Switch (Autodesk Fusion 360 design; units mm, degrees)
Autodesk Fusion 360 part; units mm, degrees
sketch "Sketch1" plane through (0, 0, 0) normal (0, 0, 1) x (1, 0, 0)
  line L0 (6.25, 9.25) -> (-6.25, 9.25)
  line L1 (-6.25, 9.25) -> (-6.25, -9.25)
  line L2 (-6.25, -9.25) -> (6.25, -9.25)
  line L3 (6.25, -9.25) -> (6.25, 9.25)
  line L4 (6.25, 9.25) -> (-6.25, -9.25) construction
  line L5 (-6.25, 9.25) -> (6.25, -9.25) construction
  dimension "d1" = 12.5
  dimension "d2" = 18.5
  constraint horizontal L0
  constraint perpendicular L0 L1
  constraint parallel L0 L2
  constraint parallel L1 L3
  constraint coincident L4 origin
  constraint coincident L5 origin
  measures "d1" distance of L1.end L2.end
  measures "d2" distance of L0.end L1.end
extrude "Extrude1" add sketch "Sketch1" along normal blind 10 makes body 1
sketch "Sketch2" plane through (0, 0, 10) normal (0, 0, 1) x (-1, 0, 0)
  line L0 (-6.25, 9.25) -> (-6.25, -9.25)
  line L1 (-6.25, -9.25) -> (6.25, -9.25)
  line L2 (6.25, -9.25) -> (6.25, 9.25)
  line L3 (6.25, 9.25) -> (-6.25, 9.25)
  line L4 (-6.5, -10) -> (6.5, -10)
  line L5 (6.5, -10) -> (6.5, 10)
  line L6 (6.5, 10) -> (-6.5, 10)
  line L7 (-6.5, 10) -> (-6.5, -10)
  line L8 (-6.5, -10) -> (6.5, 10) construction
  line L9 (6.5, -10) -> (-6.5, 10) construction
  dimension "d5" = 13
  dimension "d6" = 20
  constraint horizontal L4
  constraint perpendicular L4 L5
  constraint parallel L4 L6
  constraint parallel L5 L7
  constraint coincident L8 origin
  constraint coincident L9 origin
  measures "d5" distance of L5.end L6.end
  measures "d6" distance of L4.end L5.end
extrude "Extrude2" add sketch "Sketch2" along normal blind 4.5 contours L0 L1 L2 L3 | L4 L5 L6 L7 bodies 1
sketch "Sketch3" plane through (0, 0, 14.5) normal (0, 0, 1) x (-1, 0, 0)
  line L0 (-6.5, 10) -> (-6.5, -10)
  line L1 (-6.5, -10) -> (6.5, -10)
  line L2 (6.5, -10) -> (6.5, 10)
  line L3 (6.5, 10) -> (-6.5, 10)
  line L4 (-7.5, -10.5) -> (7.5, -10.5)
  line L5 (7.5, -10.5) -> (7.5, 10.5)
  line L6 (7.5, 10.5) -> (-7.5, 10.5)
  line L7 (-7.5, 10.5) -> (-7.5, -10.5)
  line L8 (-7.5, -10.5) -> (7.5, 10.5) construction
  line L9 (7.5, -10.5) -> (-7.5, 10.5) construction
  dimension "d9" = 15
  dimension "d10" = 21
  constraint horizontal L4
  constraint perpendicular L4 L5
  constraint parallel L4 L6
  constraint parallel L5 L7
  constraint coincident L8 origin
  constraint coincident L9 origin
  measures "d9" distance of L5.end L6.end
  measures "d10" distance of L4.end L5.end
extrude "Extrude3" add sketch "Sketch3" along normal blind 2 contours L0 L1 L2 L3 | L4 L5 L6 L7 bodies 1
sketch "Sketch4" plane through (0, 0, 16.5) normal (0, 0, 1) x (-1, 0, 0)
  line L0 (-7.5, 10.5) -> (-7.5, -10.5)
  line L1 (-7.5, -10.5) -> (7.5, -10.5)
  line L2 (7.5, -10.5) -> (7.5, 10.5)
  line L3 (7.5, 10.5) -> (-7.5, 10.5)
  line L4 (-5, -7.5) -> (5, -7.5)
  line L5 (5, -7.5) -> (5, 7.5)
  line L6 (5, 7.5) -> (-5, 7.5)
  line L7 (-5, 7.5) -> (-5, -7.5)
  line L8 (-5, -7.5) -> (5, 7.5) construction
  line L9 (5, -7.5) -> (-5, 7.5) construction
  dimension "d13" = 10
  dimension "d14" = 15
  constraint horizontal L4
  constraint perpendicular L4 L5
  constraint parallel L4 L6
  constraint parallel L5 L7
  constraint coincident L8 origin
  constraint coincident L9 origin
  measures "d13" distance of L5.end L6.end
  measures "d14" distance of L4.end L5.end
extrude "Extrude4" add sketch "Sketch4" along normal blind 3.5 contours L4 L5 L6 L7 bodies 1
sketch "Sketch5" plane through (5, 0, 0) normal (1, 0, 0) x (0, 1, 0)
  line L0 (-7.5, 16.5) -> (7.5, 16.5)
  line L1 (7.5, 16.5) -> (7.5, 20)
  line L2 (7.5, 20) -> (-7.5, 20)
  line L3 (-7.5, 20) -> (-7.5, 16.5)
  line L4 (0, 16.5) -> (7.5, 16.5)
  line L5 (0, 16.5) -> (-6.6332, 20)
  line L6 (-6.6332, 20) -> (-7.5, 16.5)
  dimension "d17" = 7.5
  constraint midpoint L0 L4.start
  constraint coincident L0.end L1.start
  constraint coincident L2 L5.end
  constraint coincident L0.start L3.end
  measures "d17" distance of L4.start L5.end
extrude "Extrude5" cut sketch "Sketch5" against normal blind 10 contours L2 L3 L6 | L0 L1 L2 L4 L5 bodies 1
sketch "Sketch6" plane through (0, 0, 16.5) normal (0, 0, 1) x (-1, 0, 0)
  line L0 (-5, 7.5) -> (5, 7.5)
  line L1 (5, 7.5) -> (5, 0)
  line L2 (5, 0) -> (-5, 0)
  line L3 (-5, 0) -> (-5, 7.5)
  line L4 (-7.5, 10.5) -> (-7.5, -10.5)
  line L5 (-7.5, -10.5) -> (7.5, -10.5)
  line L6 (7.5, -10.5) -> (7.5, 10.5)
  line L7 (7.5, 10.5) -> (-7.5, 10.5)
  line L8 (-5, -7.5) -> (5, -7.5)
  line L9 (5, -7.5) -> (5, 7.5)
  line L10 (5, 7.5) -> (-5, 7.5)
  line L11 (-5, 7.5) -> (-5, -7.5)
  line L12 (-5, -7.5) -> (5, 7.5) construction
  line L13 (5, -7.5) -> (-5, 7.5) construction
  line L14 (5.5, 8) -> (-5.5, 8)
  line L15 (-5.5, 8) -> (-5.5, -8)
  line L16 (-5.5, -8) -> (5.5, -8)
  line L17 (5.5, -8) -> (5.5, 8)
  dimension "d20" = 10
  dimension "d21" = 15
  dimension "d22" = 0.5
  constraint horizontal L8
  constraint perpendicular L8 L9
  constraint parallel L8 L10
  constraint parallel L9 L11
  constraint coincident L12 origin
  constraint coincident L13 origin
  measures "d20" distance of L0.end L0.start
  measures "d21" distance of L8.end L0.end
extrude "Extrude6" cut sketch "Sketch6" against normal blind 4 contours L14 L15 L16 L17 bodies 1
fillet "Fillet1" radius 1.5 4 edges at (7.5, -10.5, 15.5) (-7.5, -10.5, 15.5) (-7.5, 10.5, 15.5) (7.5, 10.5, 15.5) on bodies 1
fillet "Fillet2" radius 0.5 8 edges at (-7.0607, 10.0607, 16.5) (-7.5, 0, 16.5) (-7.0607, -10.0607, 16.5) (0, -10.5, 16.5) (7.0607, -10.0607, 16.5) (7.5, 0, 16.5) (7.0607, 10.0607, 16.5) (0, 10.5, 16.5) on bodies 1
fillet "Fillet3" radius 10 1 edges at (0, 0, 16.5) on bodies 1
fillet "Fillet4" radius 0.5 2 edges at (0, 7.5, 16.5) (0, -6.6332, 20) on bodies 1
fillet "Fillet5" radius 0.5 14 edges at (-5, -7.1434, 17.9399) (-5, -6.506, 19.7159) (-5, -4.1292, 18.6788) (-5, 0.0726, 16.7932) (-5, 4.7382, 16.5) (-5, 7.3536, 16.3536) (-5, 7.5, 14.25) (5, 7.5, 14.25) (5, 7.3536, 16.3536) (5, 4.7382, 16.5) (5, 0.0726, 16.7932) (5, -4.1292, 18.6788) (5, -6.506, 19.7159) (5, -7.1434, 17.9399) on bodies 1
sketch "Sketch7" plane through (0, 0, 16.5) normal (0, 0, 1) x (-1, 0, 0)
  line L0 (-4.5, -2.4764) -> (-4.5, -7)
  line L1 (-4.5, -7) -> (4.5, -7)
  line L2 (4.5, -7) -> (4.5, -2.4764)
  line L3 (4.5, -2.4764) -> (-4.5, -2.4764)
  line L4 (-4.5, -7) -> (4.5, -2.4764) construction
  circle A0 centre (0, -4.7382) radius 1.5
  dimension "d35" = 3
  constraint coincident L0.end L1.start
  constraint coincident L2.end L3.start
  constraint midpoint L4 A0.centre
  measures "d35" diameter of A0
extrude "Extrude7" add sketch "Sketch7" along normal blind 0.5 draft -45 contours A0 bodies 1
fillet "Fillet6" radius 0.5 1 edges at (0.9323, 4.3766, 17) on bodies 1
sketch "Sketch8" plane through (0, 0, 0) normal (0, 0, -1) x (1, 0, 0)
  line L0 (6.25, -9.25) -> (6.25, 9.25)
  line L1 (6.25, 9.25) -> (-6.25, 9.25)
  line L2 (-6.25, 9.25) -> (-6.25, -9.25)
  line L3 (-6.25, -9.25) -> (6.25, -9.25)
  line L4 (2.5, 7.5) -> (-2.5, 7.5) construction
  line L5 (-2.5, 7.5) -> (-2.5, -7.5) construction
  line L6 (-2.5, -7.5) -> (2.5, -7.5) construction
  line L7 (2.5, -7.5) -> (2.5, 7.5) construction
  line L8 (2.5, 7.5) -> (-2.5, -7.5) construction
  line L9 (-2.5, 7.5) -> (2.5, -7.5) construction
  line L10 (-2.5, 7.5) -> (2.5, 7.5)
  line L11 (2.5, 7.5) -> (2.5, 6.5)
  line L12 (2.5, 6.5) -> (-2.5, 6.5)
  line L13 (-2.5, 6.5) -> (-2.5, 7.5)
  line L14 (-2.5, -7.5) -> (2.5, -7.5)
  line L15 (2.5, -7.5) -> (2.5, -6.5)
  line L16 (2.5, -6.5) -> (-2.5, -6.5)
  line L17 (-2.5, -6.5) -> (-2.5, -7.5)
  line L18 (2.5, 0.5) -> (-2.5, 0.5)
  line L19 (-2.5, 0.5) -> (-2.5, -0.5)
  line L20 (-2.5, -0.5) -> (2.5, -0.5)
  line L21 (2.5, -0.5) -> (2.5, 0.5)
  line L22 (2.5, 0.5) -> (-2.5, -0.5) construction
  line L23 (-2.5, 0.5) -> (2.5, -0.5) construction
  dimension "d40" = 5
  dimension "d41" = 15
  dimension "d42" = 5
  dimension "d43" = 1
  dimension "d44" = 5
  dimension "d45" = 1
  dimension "d46" = 5
  dimension "d47" = 1
  constraint horizontal L4
  constraint perpendicular L4 L5
  constraint parallel L4 L6
  constraint parallel L5 L7
  constraint coincident L8 origin
  constraint coincident L9 origin
  constraint horizontal L10
  constraint vertical L11
  constraint horizontal L12
  constraint vertical L13
  constraint horizontal L14
  constraint vertical L15
  constraint horizontal L16
  constraint vertical L17
  constraint horizontal L18
  constraint perpendicular L18 L19
  constraint parallel L18 L20
  constraint parallel L19 L21
  constraint coincident L22 origin
  constraint coincident L23 origin
  measures "d40" distance of L5.end L6.end
  measures "d41" distance of L4.end L5.end
  measures "d42" distance of L4.end L4.start
  measures "d43" distance of L4.end L12.end
  measures "d44" distance of L5.end L6.end
  measures "d45" distance of L5.end L16.end
  measures "d46" distance of L19.end L20.end
  measures "d47" distance of L18.end L19.end
extrude "Extrude8" add sketch "Sketch8" along normal blind 7 separate body contours L10 L11 L12 L13 | L14 L15 L16 L17 | L18 L19 L20 L21 makes body 2 at (0.8333, 6.5, -2.3333) makes body 3 at (-0.8333, 0.5, -2.3333) makes body 4 at (-0.8333, -7.5, -2.3333)
sketch "Sketch9" plane through (0, 7.5, 0) normal (0, 1, 0) x (-1, 0, 0)
  line L0 (2.5, 0) -> (-2.5, 0)
  line L1 (-2.5, 0) -> (-2.5, -7)
  line L2 (-2.5, -7) -> (2.5, -7)
  line L3 (2.5, -7) -> (2.5, 0)
  line L4 (0, -7) -> (0, -4)
  circle A0 centre (0, -4) radius 1
  dimension "d50" = 3
  dimension "d51" = 2
  constraint midpoint L2 L4.start
  constraint perpendicular L2 L4
  constraint coincident L4.end A0.centre
  measures "d50" distance of L4.start L4.end
  measures "d51" diameter of A0
extrude "Extrude9" cut sketch "Sketch9" against normal blind 15 contours A0 bodies 2 3 4
chamfer "Chamfer1" distance 1 angle 45 6 edges at (2.5, -7, -7) (-2.5, -7, -7) (2.5, 0, -7) (-2.5, 0, -7) (2.5, 7, -7) (-2.5, 7, -7) on bodies 2 3 4
combine "Combine1" operation add target body 1 tool bodies 2 3 4
